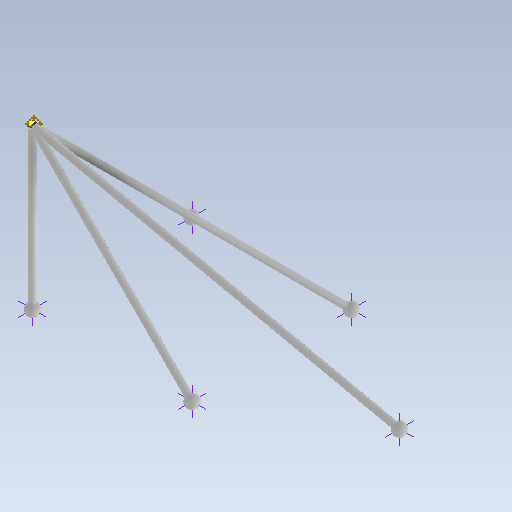
# Autodesk Inventor part: Coupler
Saved by Autodesk Inventor 2020.1 (Build 241239000, 239)
## iProperties
Created: 2019-10-25
Part Number: Coupler
Material: Generic
Document SubType Name: Modeling
Designer: sshel
Density: 1 g/cm^3
Appearance: Default
Mass: 10990.7 g
Surface Area: 10781.2 cm^2
Volume: 10990.7 cm^3
Author: sshel
Autodesk Inventor part; units mm, degrees
ref_plane "Dyad1 plane" through (0, 0, -1000) normal (0, 0, -1) x (-1, 0, 0)
sketch "Sketch3" plane through (0, 0, -1000) normal (0, 0, -1) x (-1, 0, 0)
  circle A0 centre (0, 0) radius 20
  dimension "d16" = 20
  constraints: 1 centre point, 1 coincident
  measures "d16" radius of A0
sketch3d "import_point_3Dsketch"
  line L0 (0, 0, -1000) -> (0, 0, 0)
sweep "Dyad1 rod" add profiles "Sketch3" path "import_point_3Dsketch"
sketch "Sketch2" plane through (0, 0, -1000) normal (0, 0, -1) x (-1, 0, 0)
  circle A0 centre (0, 0) radius 40
  line L0 (40, 0) -> (-40, 0)
  dimension "d17" = 40
  constraints: 2 end point, 2 point on circle, 1 centre point, 1 coincident, 1 horizontal, 1 midpoint
  measures "d17" radius of A0
revolve "Dyad1 joint" add sketch "Sketch2" angle 360 about axis through (-40, 0, -1000) along (1, 0, 0) separate body picked at (-4.1202, -12.6808) contours A0 L0
ref_plane "Dyad2 plane" through (1000, 0, -1000) normal (0.7071068, 0, -0.7071068) x (0, 1, 0)
sketch "Sketch4" plane through (1000, 0, -1000) normal (0.7071068, 0, -0.7071068) x (0, 1, 0)
  circle A0 centre (0, 0) radius 20
  dimension "d14" = 20
  constraints: 1 centre point, 1 coincident
  measures "d14" radius of A0
sketch3d "import_point_3Dsketch for Dyad2 rod"
  line L0 (1000, 0, -1000) -> (0, 0, 0)
sweep "Dyad2 rod" add profiles "Sketch4" path "import_point_3Dsketch for Dyad2 rod" separate body
sketch "Sketch5" plane through (1000, 0, -1000) normal (0.7071068, 0, -0.7071068) x (0, 1, 0)
  circle A0 centre (0, 0) radius 40
  line L0 (40, 0) -> (-40, 0)
  dimension "d11" = 40
  constraints: 2 end point, 2 point on circle, 1 centre point, 1 coincident, 1 horizontal, 1 midpoint
  measures "d11" radius of A0
revolve "Dyad2 joint" add sketch "Sketch5" angle 360 about axis through (1000, 40, -1000) along (0, -1, 0) picked at (-4.1202, -12.6808) bodies 2 contours A0 L0
ref_plane "Dyad3 plane" through (0, 1000, -1000) normal (0, 0.7071068, -0.7071068) x (-1, 0, 0)
sketch "Sketch6" plane through (0, 1000, -1000) normal (0, 0.7071068, -0.7071068) x (-1, 0, 0)
  circle A0 centre (0, 0) radius 20
  dimension "d18" = 20
  constraints: 1 centre point, 1 coincident
  measures "d18" radius of A0
sketch3d "import_point_3Dsketch for Dyad3 rod"
  line L0 (0, 1000, -1000) -> (0, 0, 0)
sweep "Dyad3 rod" add profiles "Sketch6" path "import_point_3Dsketch for Dyad3 rod" separate body
sketch "Sketch7" plane through (0, 1000, -1000) normal (0, 0.7071068, -0.7071068) x (-1, 0, 0)
  circle A0 centre (0, 0) radius 40
  line L0 (40, 0) -> (-40, 0)
  dimension "d21" = 40
  constraints: 2 end point, 2 point on circle, 1 centre point, 1 coincident, 1 horizontal, 1 midpoint
  measures "d21" radius of A0
revolve "Dyad3 joint" add sketch "Sketch7" angle 360 about axis through (-40, 1000, -1000) along (1, 0, 0) picked at (-4.1202, -12.6808) bodies 2 contours A0 L0
ref_plane "Dyad4 plane" through (1000, 1000, -1000) normal (0.5773503, 0.5773503, -0.5773503) x (-0.7071068, 0.7071068, 0)
sketch "Sketch8" plane through (1000, 1000, -1000) normal (0.5773503, 0.5773503, -0.5773503) x (-0.7071068, 0.7071068, 0)
  circle A0 centre (0, 0) radius 20
  dimension "d23" = 20
  constraints: 1 centre point, 1 coincident
  measures "d23" radius of A0
sketch3d "import_point_3Dsketch for Dyad4 rod"
  line L0 (1000, 1000, -1000) -> (0, 0, 0)
sweep "Dyad4 rod" add profiles "Sketch8" path "import_point_3Dsketch for Dyad4 rod" separate body
sketch "Sketch9" plane through (1000, 1000, -1000) normal (0.5773503, 0.5773503, -0.5773503) x (-0.7071068, 0.7071068, 0)
  circle A0 centre (0, 0) radius 40
  line L0 (40, 0) -> (-40, 0)
  dimension "d26" = 40
  constraints: 2 end point, 2 point on circle, 1 centre point, 1 coincident, 1 horizontal, 1 midpoint
  measures "d26" radius of A0
revolve "Dyad4 joint" add sketch "Sketch9" angle 360 about axis through (971.7157, 1028.2843, -1000) along (0.7071068, -0.7071068, 0) picked at (-4.1202, -12.6808) bodies 2 contours A0 L0
ref_plane "Dyad5 plane" through (1800, 500, -1000) normal (0.8494725, 0.2359646, -0.4719292) x (-0.2676439, 0.9635179, 0)
sketch "Sketch10" plane through (1800, 500, -1000) normal (0.8494725, 0.2359646, -0.4719292) x (-0.2676439, 0.9635179, 0)
  circle A0 centre (0, 0) radius 20
  point P0 (0, 0)
  dimension "d28" = 20
  constraints: 1 centre point, 1 coincident
  measures "d28" radius of A0
sketch3d "import_point_3Dsketch for Dyad5 rod"
  line L0 (1800, 500, -1000) -> (0, 0, 0)
sweep "Dyad5 rod" add profiles "Sketch10" path "import_point_3Dsketch for Dyad5 rod" separate body
sketch "Sketch11" plane through (1800, 500, -1000) normal (0.8494725, 0.2359646, -0.4719292) x (-0.2676439, 0.9635179, 0)
  circle A0 centre (0, 0) radius 40
  line L0 (40, 0) -> (-40, 0)
  point P0 (0, 0)
  dimension "d31" = 40
  constraints: 2 end point, 2 point on circle, 1 centre point, 1 coincident, 1 horizontal, 1 midpoint
  measures "d31" radius of A0
revolve "Dyad5 joint" add sketch "Sketch11" angle 360 about axis through (1789.2942, 538.5407, -1000) along (0.2676439, -0.9635179, 0) picked at (-4.1202, -12.6808) bodies 2 contours A0 L0
equation "\"d16\" = rod_radius"
equation "\"d17\" = S_radius"
equation "\"d14\" = rod_radius"
equation "\"d11\" = S_radius"
equation "\"d18\" = rod_radius"
equation "\"d21\" = S_radius"
equation "\"d23\" = rod_radius"
equation "\"d26\" = S_radius"
equation "\"d28\" = rod_radius"
equation "\"d31\" = S_radius"
equation "\"rod_radius\" = 20"
equation "\"S_radius\" = 2 * rod_radius"
body "Solid2"
body "Solid3"
body "Solid4"
body "Solid5"
body "Solid6"
body "Solid7"
